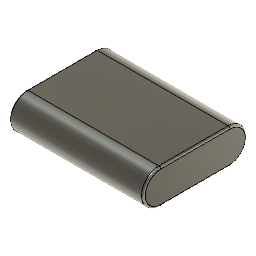
353 6600mAh Battery (Autodesk Fusion 360 design; units mm, degrees)
Autodesk Fusion 360 part; units mm, degrees
sketch "Sketch2" plane through (0, 0, 0) normal (0, 0, 1) x (1, 0, 0)
  line L0 (0, 0) -> (70, 0)
  line L1 (70, 0) -> (70, 54)
  line L2 (70, 54) -> (0, 54)
  line L3 (0, 54) -> (0, 0)
  dimension "d72" = 70
  dimension "d73" = 54
  measures "d72" distance of L0.start L0.end
  measures "d73" distance of L0.start L2.end
extrude "Extrude1" add sketch "Sketch2" along normal blind 18
fillet "Fillet1" radius 9 4 edges at (35, 54, 18) (35, 54, 0) (35, 0, 18) (35, 0, 0)
fillet "Fillet2" radius 1 8 edges at (0, 27, 0) (0, 54, 9) (0, 27, 18) (0, 0, 9) (70, 27, 0) (70, 0, 9) (70, 27, 18) (70, 54, 9)
